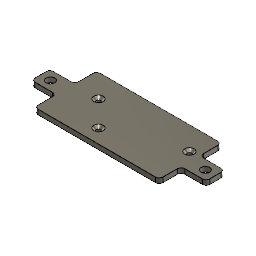
Sonar PCB Bracket v1 (Autodesk Fusion 360 design; units mm, degrees)
Autodesk Fusion 360 part; units mm, degrees
sketch "Sketch1" plane through (0, 0, 0) normal (0, 1, 0) x (1, 0, 0)
  line L0 (50, 25) -> (-50, 25)
  line L1 (-50, 25) -> (-50, -25)
  line L2 (-50, -25) -> (50, -25)
  line L3 (50, -25) -> (50, 25)
  line L4 (50, 25) -> (-50, -25) construction
  line L5 (-50, 25) -> (50, -25) construction
  line L6 (0, 0) -> (0, 15) construction
  line L7 (0, 0) -> (-17.4892, 0) construction
  circle A0 centre (42.83, 6.35) radius 1.75
  circle A1 centre (-30, 6.35) radius 1.75
  circle A2 centre (-9.85, -13.8) radius 1.75
  line L8 (70, 7.5) -> (50, 7.5)
  line L9 (50, 7.5) -> (50, -7.5)
  line L10 (50, -7.5) -> (70, -7.5)
  line L11 (70, -7.5) -> (70, 7.5)
  line L12 (70, 7.5) -> (50, -7.5) construction
  line L13 (50, 7.5) -> (70, -7.5) construction
  line L14 (-70, 7.5) -> (-50, 7.5)
  line L15 (-70, -7.5) -> (-70, 7.5)
  line L16 (-50, -7.5) -> (-70, -7.5)
  circle A3 centre (62, 0) radius 3.4
  circle A4 centre (-62, 0) radius 3.4
  line L17 (42.83, 6.35) -> (-30, 6.35) construction
  point P0 (60, 0)
  dimension "d1" = 3.5
  dimension "d2" = 3.5
  dimension "d3" = 3.5
  dimension "d4" = 6.8
  dimension "d5" = 15
  dimension "d6" = 20
  dimension "d7" = 12
  dimension "d8" = 100
  dimension "d9" = 50
  dimension "d10" = 72.83
  dimension "d11" = 20.15
  dimension "d12" = 20.15
  dimension "d13" = 20
  dimension "d14" = 18.65
  constraint perpendicular L0 L1
  constraint parallel L0 L2
  constraint parallel L1 L3
  constraint horizontal L0
  constraint coincident L4 L6.start
  constraint coincident L5 L6.start
  constraint coincident L6.start L7.start
  constraint vertical L6
  constraint perpendicular L6 L7
  constraint perpendicular L8 L9
  constraint parallel L8 L10
  constraint parallel L9 L11
  constraint horizontal L8
  constraint coincident L12 P0
  constraint coincident L13 P0
  constraint coincident L7 P0
  constraint collinear L3 L9
  constraint symmetric L6 L8.start L14.start
  constraint symmetric L6 L8.end L14.end
  constraint symmetric L6 L9.end L16.start
  constraint symmetric L6 L10.end L15.start
  constraint coincident L7 A3.centre
  constraint symmetric L6 A3 A4
  constraint coincident A0.centre L17.start
  constraint coincident A1.centre L17.end
  constraint horizontal L17
  measures "d1" diameter of A2
  measures "d2" diameter of A1
  measures "d3" diameter of A0
  measures "d4" diameter of A3
  measures "d5" distance of L8.start L10.end
  measures "d6" distance of L8.start L8.end
  measures "d7" distance of L3 A3.centre
  measures "d8" distance of L0.start L0.end
  measures "d9" distance of L0.start L2.end
  measures "d10" horizontal distance of A0.centre A1.centre
  measures "d11" vertical distance of A1.centre A2.centre
  measures "d12" horizontal distance of A1.centre A2.centre
  measures "d13" distance of L1 A1.centre
  measures "d14" distance of L0 A1.centre
extrude "Extrude1" add sketch "Sketch1" along normal blind 4
fillet "Fillet1" radius 3 12 edges at (50, 2, 7.5) (50, 2, 25) (70, 2, 7.5) (70, 2, -7.5) (50, 2, -7.5) (50, 2, -25) (-50, 2, -25) (-50, 2, -7.5) (-70, 2, -7.5) (-70, 2, 7.5) (-50, 2, 7.5) (-50, 2, 25)
chamfer "Chamfer1" distance 2 angle 45 3 edges at (41.1984, 4, -6.9828) (-11.4816, 4, 13.1672) (-31.6316, 4, -6.9828)
